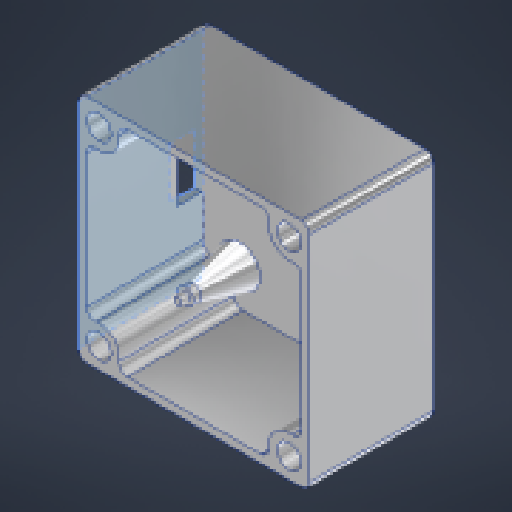
# Autodesk Inventor part: ELP Camera Case
Saved by Autodesk Inventor 2023.3 (Build 273359000, 359)
## iProperties
Created: 2024-02-12
Part Number: ELP Camera Case
Material: Aluminum 6061
Document SubType Name: Modeling
Designer: mavericks
Density: 2.7 g/cm^3
Appearance: Aluminum - Flat
Author: mavericks
Autodesk Inventor part; units mm, degrees
ref_plane "YZ Plane" through (0, 0, 0) normal (1, 0, 0) x (0, 1, 0)
ref_plane "XZ Plane" through (0, 0, 0) normal (0, 1, 0) x (-1, 0, 0)
ref_plane "XY Plane" through (0, 0, 0) normal (0, 0, 1) x (1, 0, 0)
sketch "Sketch1" plane through (0, 0, 0) normal (0, 0, 1) x (1, 0, 0)
  line L0 (-19, 19) -> (19, 19) construction
  line L1 (19, 19) -> (19, -19) construction
  line L2 (19, -19) -> (-19, -19) construction
  line L3 (-19, -19) -> (-19, 19) construction
  line L4 (-19, 19) -> (19, -19) construction
  line L5 (19, 19) -> (-19, -19) construction
  line L6 (-17, 17) -> (17, 17) construction
  line L7 (17, 17) -> (17, -17) construction
  line L8 (17, -17) -> (-17, -17) construction
  line L9 (-17, -17) -> (-17, 17) construction
  line L10 (-17, 17) -> (17, -17) construction
  line L11 (17, 17) -> (-17, -17) construction
  line L12 (28, 28) -> (-28, 28)
  line L13 (-28, 28) -> (-28, -28)
  line L14 (-28, -28) -> (28, -28)
  line L15 (28, -28) -> (28, 28)
  circle A0 centre (-23, 23) radius 5 construction
  circle A1 centre (23, 23) radius 5 construction
  line L16 (23, -23) -> (-23, -23) construction
  line L17 (-23, -23) -> (-23, 23) construction
  line L18 (-23, 23) -> (23, 23) construction
  line L19 (23, 23) -> (23, -23) construction
  line L20 (23, -23) -> (-23, 23) construction
  line L21 (-23, -23) -> (23, 23) construction
  circle A2 centre (-17, 17) radius 2
  circle A3 centre (17, 17) radius 2
  circle A4 centre (17, -17) radius 2
  circle A5 centre (-17, -17) radius 2
  point P0 (0, 0)
  dimension "d0" = 38
  dimension "d1" = 38
  dimension "d2" = 34
  dimension "d3" = 34
  dimension "d8" = 10
  dimension "d9" = 46
  dimension "d18" = 4
  dimension "d19" = 4
  dimension "d20" = 4
  dimension "d21" = 4
  constraints: 44 end point, 11 coincident, 8 parallel, 6 centre point, 6 midpoint, 4 perpendicular, 4 tangent, 3 horizontal, 2 point on line, 1 equal radius, 3 other
  measures "d0" distance of L1.end L2.end
  measures "d1" distance of L0.end L1.end
  measures "d2" distance of L7.end L8.end
  measures "d3" distance of L6.end L7.end
  measures "d8" diameter of A0
  measures "d9" distance of A1.centre L17.end
  measures "d18" diameter of A2
  measures "d19" diameter of A3
  measures "d20" diameter of A4
  measures "d21" diameter of A5
extrude "Extrusion1" add sketch "Sketch1" along normal blind 30 contours L15 L14 L13 L12 | A2 | A3 | A4 | A5
hole "Hole1" at (23, 23, 0) at (-23, 23, 0) at (-23, -23, 0) at (23, -23, 0) direction (0, 0, 1) diameter 5.8 end through all
shell "Shell1" thickness 2 removed faces 1 at (7.0256, -6.9431, 30)
fillet "Fillet1" radius 2 12 edges at (-26, -19.1257, 16) (-19.1257, -26, 16) (-19.1257, 26, 16) (-26, 19.1257, 16) (19.1257, 26, 16) (26, 19.1257, 16) (26, -19.1257, 16) (19.1257, -26, 16) (28, -28, 15) (-28, -28, 15) (-28, 28, 15) (28, 28, 15)
extrude "Extrusion2" add sketch "Sketch1" along normal blind 15 contours A2 | A3 | A4 | A5
chamfer "Chamfer1" distance 3 angle 75 4 edges at (-19, 17, 2) (15, 17, 2) (15, -17, 2) (-19, -17, 2) measured on face at (14.5, 17, 2) measured on face at (-19.5, 17, 2) measured on face at (14.5, -17, 2) measured on face at (-19.5, -17, 2)
sketch "Sketch2" plane through (-17, 17, 15) normal (0, 0, 1) x (1, 0, 0)
  circle A0 centre (0, 0) radius 2 construction
  circle A1 centre (0, 0) radius 0.95
  circle A2 centre (34, 0) radius 2 construction
  circle A3 centre (34, -34) radius 2 construction
  circle A4 centre (0, -34) radius 2 construction
  circle A5 centre (34, 0) radius 0.95
  circle A6 centre (34, -34) radius 2 construction
  circle A7 centre (34, -34) radius 0.95
  circle A8 centre (0, -34) radius 0.95
  point P0 (17, -17)
  dimension "d27" = 1.9
  dimension "d28" = 1.9
  dimension "d29" = 1.9
  dimension "d30" = 1.9
  constraints: 4 centre point, 4 coincident
  measures "d27" diameter of A1
  measures "d28" diameter of A5
  measures "d29" diameter of A7
  measures "d30" diameter of A8
extrude "Extrusion3" add sketch "Sketch2" along normal blind 2
sketch "Sketch3" plane through (0, 0, 0) normal (0, 0, -1) x (-1, 0, 0)
  point P0 (0, 0)
sketch "Sketch4" plane through (-28, -26, 0) normal (-1, 0, 0) x (0, 0, 1)
  line L0 (2, 20) -> (8, 20)
  line L1 (8, 20) -> (8, 32)
  line L2 (8, 32) -> (2, 32)
  line L3 (2, 32) -> (2, 20)
  line L4 (2, 20) -> (8, 32) construction
  line L5 (8, 20) -> (2, 32) construction
  line L6 (0, 52) -> (0, 0) construction
  point P0 (0, 26)
  point P1 (5, 26)
  point P2 (0, 26)
  dimension "d33" = 12
  dimension "d34" = 6
  dimension "d35" = 2
  constraints: 12 end point, 3 midpoint, 2 parallel, 1 horizontal, 1 horizontal alignment, 1 perpendicular
  measures "d33" distance of L2.end L0.start
  measures "d34" distance of L1.end L2.end
  measures "d35" distance between parallel lines of L3 L6
extrude "Extrusion4" cut sketch "Sketch4" against normal up to next
ref_plane "Work Plane1" through (-26, 3.75, 0) normal (0, -1, 0) x (1, 0, 0)
sketch "Sketch5" plane through (-26, 3.75, 0) normal (0, -1, 0) x (1, 0, 0)
  line L0 (0, 8) -> (-2, 8) construction
  line L1 (-2, 8) -> (-2, 30) construction
  line L2 (-2, 30) -> (0, 30) construction
  line L3 (0, 30) -> (0, 8) construction
  line L4 (54, 30) -> (54, 0) construction
  line L5 (54, 0) -> (-2, 0) construction
  line L6 (-2, 0) -> (-2, 2) construction
  line L7 (-2, 2) -> (52, 2) construction
  line L8 (52, 2) -> (52, 30) construction
  line L9 (52, 30) -> (54, 30) construction
  line L10 (19.3594, 2) -> (21.5729, 4.2135)
  line L11 (21.5729, 4.2135) -> (26.5729, 4.2135)
  line L12 (42.1728, 2) -> (9.8272, 2) construction
  line L13 (26.5729, 4.2135) -> (28.7865, 2)
  line L14 (16.531, 2) -> (31.6149, 2)
  line L15 (16.531, 2) -> (20.7445, 6.2135)
  line L16 (20.7445, 6.2135) -> (27.4014, 6.2135)
  line L17 (27.4014, 6.2135) -> (31.6149, 2)
  point P0 (26, 0)
  dimension "d39" = 45
  dimension "d40" = 5
  dimension "d41" = 2
  constraints: 14 end point, 6 point on line, 2 perpendicular, 1 collinear, 1 parallel
  measures "d39" angle of L7 L10
  measures "d40" distance of L10.end L11.end
  measures "d41" distance between parallel lines of L10 L15
extrude "Extrusion5" add sketch "Sketch5" against normal blind 5 contours L14 L15 L16 L17 L13 L11 L10
chamfer "Chamfer2" distance 0.5 angle 45 12 edges at (-1.9271, 3.75, 6.2135) (-1.9271, 3.75, 4.2135) (1.6797, 3.75, 3.1068) (3.5081, 3.75, 4.1068) (3.5081, 8.75, 4.1068) (-7.3623, 3.75, 4.1068) (-5.5338, 3.75, 3.1068) (-7.3623, 8.75, 4.1068) (-5.5338, 8.75, 3.1068) (1.6797, 8.75, 3.1068) (-1.9271, 8.75, 4.2135) (-1.9271, 8.75, 6.2135)
body "Solid1"
